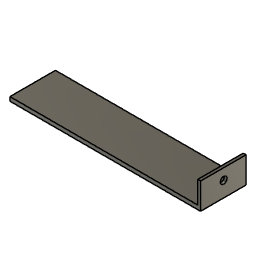
Antenna L Bracket v2 (Autodesk Fusion 360 design; units mm, degrees)
Autodesk Fusion 360 part; units mm, degrees
box "BoxPrimitive1" add length 40 width 165 height 3.5 placed x (0, 1, 0) y (-1, 0, 0) z (0, 0, 1) at (165, 0, 0)
box "BoxPrimitive2" add length 40 width 2.5 height 23 placed x (0, 1, 0) y (-1, 0, 0) z (0, 0, 1) at (167.5, 0, 0)
hole "Hole1" at (167.5, 20.3218, 13.4545) direction (-1, 0, 0) diameter 6 depth 5 tip angle 180
